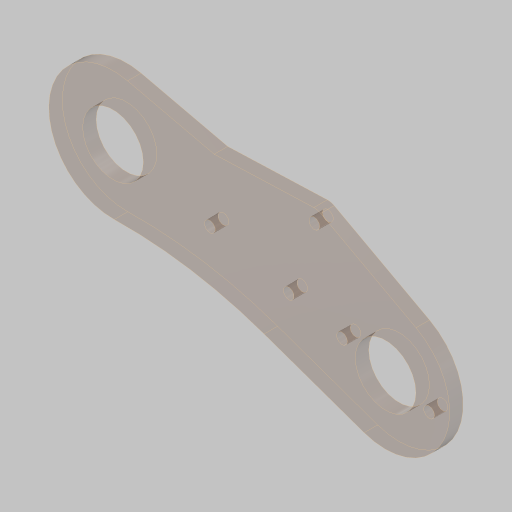
# Autodesk Inventor part: GP10-002
Saved by Autodesk Inventor 2023.5 (Build 275446000, 446)
## iProperties
Created: 2025-02-24
Part Number: GP10-002
Material: Polycarbonate, Smoke
Document SubType Name: Modeling
Designer: dlangdon
Density: 1.2 g/cm^3
Appearance: Polycarbonate - Smoked
Author: dlangdon
Autodesk Inventor part; units mm, degrees
ref_plane "YZ Plane" through (0, 0, 0) normal (1, 0, 0) x (0, 1, 0)
ref_plane "XZ Plane" through (0, 0, 0) normal (0, 1, 0) x (-1, 0, 0)
ref_plane "XY Plane" through (0, 0, 0) normal (0, 0, 1) x (1, 0, 0)
sketch "Sketch1" plane through (0, 0, 0) normal (0, 0, 1) x (1, 0, 0)
  circle A0 centre (71.842, 71.842) radius 50.8 construction
  circle A1 centre (-71.842, -71.842) radius 50.8 construction
  circle A2 centre (0, 0) radius 50.8 construction
  line L0 (-35.921, -35.921) -> (35.921, 35.921) construction
  line L1 (71.842, 71.842) -> (-71.842, -71.842) construction
  line L2 (-4.3707, 6.2419) -> (-4.3707, 50.6116) construction
  line L3 (-226.8798, -122.642) -> (638.5123, -122.642) construction
  circle A3 centre (147.8406, -65.492) radius 57.15 construction
  circle A4 centre (71.842, 71.842) radius 14.2621
  circle A5 centre (-71.842, -71.842) radius 14.2621
  circle A6 centre (-4.3707, 6.2419) radius 57.15 construction
  circle A7 centre (-71.842, -71.842) radius 30.1371 construction
  circle A8 centre (71.842, 71.842) radius 30.1371 construction
  circle A9 centre (-56.3286, 101.6778) radius 14.2621
  line L4 (-56.3286, 101.6778) -> (71.842, 71.842) construction
  circle A10 centre (71.842, 71.842) radius 14.3256 construction
  circle A11 centre (-71.842, -71.842) radius 14.3256 construction
  circle A12 centre (-78.675, 59.5778) radius 14.2621
  line L5 (-71.842, -71.842) -> (-78.675, 59.5778) construction
  circle A13 centre (-78.675, 59.5778) radius 23.8316 construction
  circle A14 centre (-56.3286, 101.6778) radius 23.8316 construction
  line L6 (14.7165, 60.1103) -> (61.7767, 43.4355)
  line L7 (-43.0113, -63.0652) -> (-59.0434, -10.4018)
  arc A15 (14.7165, 60.1103) -> (-59.0434, -10.4018) centre (-4.3707, 6.2419) ccw
  line L8 (-202.9564, 165.4321) -> (-177.9423, 161.0215)
  line L9 (-177.9423, 161.0215) -> (-204.4062, 10.9368) construction
  line L10 (-204.4062, 10.9368) -> (-229.4204, 15.3474) construction
  line L11 (-229.4204, 15.3474) -> (-202.9564, 165.4321) construction
  line L12 (-248.4004, -92.2937) -> (35.0702, -142.2772) construction
  line L13 (-201.8537, 171.6857) -> (161.0026, 107.7043) construction
  line L14 (-201.8537, 171.6857) -> (-248.4004, -92.2937) construction
  circle A16 centre (-147.7392, 94.6182) radius 31.75 construction
  line L15 (-77.4376, 35.7784) -> (-74.4797, -21.1106) construction
  line L16 (-190.4493, 163.2268) -> (-216.9133, 13.1421) construction
  line L17 (-193.206, 147.593) -> (-214.1566, 28.7759) construction
  circle A17 centre (-147.7392, 94.6182) radius 17.4625 construction
  circle A18 centre (-147.7392, 94.6182) radius 9.525
  circle A19 centre (-56.3286, 101.6778) radius 30.1816 construction
  line L18 (-202.9564, 165.4321) -> (-229.4204, 15.3474)
  arc A20 (61.7767, 43.4355) -> (78.6846, 101.1921) centre (71.842, 71.842) ccw
  arc A21 (-99.1524, -84.5852) -> (-43.0113, -63.0652) centre (-71.842, -71.842) ccw
  line L19 (-147.7392, 94.6182) -> (-131.3298, 100.5908) construction
  line L20 (-113.4287, 107.1063) -> (-182.0497, 82.1302) construction
  circle A22 centre (-182.0497, 82.1302) radius 4.7625 construction
  line L21 (0, 0) -> (-4.3707, 6.2419) construction
  circle A23 centre (71.842, 71.842) radius 28.6512 construction
  line L22 (62.334, 44.8145) -> (-61.0615, 88.2239) construction
  line L23 (75.2477, 100.2901) -> (-54.6333, 115.8388) construction
  line L24 (-177.9423, 161.0215) -> (78.6846, 101.1921)
  line L25 (-147.7392, 94.6182) -> (-125.7265, 22.8485) construction
  circle A24 centre (-125.7265, 22.8485) radius 31.75 construction
  circle A25 centre (-125.7265, 22.8485) radius 14.2621
  line L26 (-78.675, 59.5778) -> (-125.7265, 22.8485) construction
  circle A26 centre (-147.7392, 94.6182) radius 25.4 construction
  arc A27 (-99.1524, -84.5852) -> (-229.4204, 15.3474) centre (-260.2996, -159.7777) ccw
  circle A28 centre (-147.7392, 94.6182) radius 36.5125 construction
  line L27 (-180.8308, 110.0491) -> (-147.7392, 94.6182) construction
  arc A29 (-39.1085, 126.4648) -> (-49.6289, 131.1064) centre (-56.3286, 101.6778) ccw
  arc A30 (-38.1634, 52.3307) -> (-39.1085, 126.4648) centre (-65.0941, 89.0604) ccw
  arc A31 (14.7165, 60.1103) -> (-55.7287, 71.5022) centre (-51.7719, -127.535) ccw
  arc A32 (-49.6289, 131.1064) -> (-55.7287, 71.5022) centre (-56.3286, 101.6778) ccw
  line L28 (-10.7972, 91.0789) -> (26.3107, 82.4409) construction
  point P0 (-75.9587, 7.3339)
  point P1 (-203.6813, 88.1845)
  point P2 (-203.6813, 88.1845)
  point P3 (-144.7069, 111.8154)
  point P4 (-161.1163, 105.8429)
  point P5 (-164.1486, 88.6457)
  point P6 (-150.7715, 77.421)
  point P7 (-134.3622, 83.3936)
  point P8 (-123.871, 103.3056)
  point P9 (-143.3285, 119.6324)
  point P10 (-167.1967, 110.945)
  point P11 (-171.6074, 85.9309)
  point P12 (-152.1499, 69.6041)
  point P13 (-128.2817, 78.2914)
  point P14 (-160.2272, 128.9288)
  point P15 (-182.0497, 82.1302)
  point P16 (-135.2512, 60.3077)
  point P17 (-132.3084, 127.7098)
  point P18 (-163.1701, 61.5267)
  point P19 (-114.6476, 79.1874)
  point P20 (-49.4759, 131.0711)
  point P21 (7.7567, 86.7599)
  dimension "d7" = 101.6
  dimension "d18" = 47.6631
  dimension "d34" = 34.925
  dimension "d65" = 50.8
  dimension "d3" = 45
  dimension "d4" = 0
  dimension "d8" = 101.6
  dimension "d9" = 28.5242
  dimension "d10" = 101.6
  dimension "d11" = 114.3
  dimension "d12" = 114.3
  dimension "d13" = 15.875
  dimension "d14" = 15.875
  dimension "d15" = 131.5974
  dimension "d16" = 28.6512
  dimension "d17" = 131.5974
  dimension "d19" = 47.6631
  dimension "d22" = 25.4
  dimension "d23" = 152.4
  dimension "d26" = 268.0517
  dimension "d27" = 63.5
  dimension "d30" = 203.2
  dimension "d31" = 10
  dimension "d33" = 120.65
  dimension "d35" = 19.05
  dimension "d36" = 6.35
  dimension "d40" = 360
  dimension "d44" = 9.525
  dimension "d55" = 80
  dimension "d56" = 7.62
  dimension "d57" = 6.35
  dimension "d58" = 57.3024
  dimension "d59" = 63.5
  dimension "d60" = 75.0697
  dimension "d61" = 59.69
  dimension "d62" = 55
  dimension "d68" = 360
  dimension "d70" = 41.275
  dimension "d71" = 60
  dimension "d82" = 360
  dimension "d87" = 360
  dimension "d89" = 45
  dimension "d105" = 38.1
  constraints: 58 end point, 34 point on circle, 29 centre point, 27 coincident, 19 tangent, 9 midpoint, 6 equal radius, 6 point on line, 4 collinear, 4 parallel, 2 horizontal, 1 concentric, 1 perpendicular, 1 vertical, 39 other
  measures "d3" angle of L2 L0
  measures "d4" distance between parallel lines of L0 L1
  measures "d8" diameter of A2
  measures "d9" diameter of A4
  measures "d10" diameter of A0
  measures "d11" diameter of A3
  measures "d12" diameter of A6
  measures "d13" radial gap between concentric circles of A5 A7
  measures "d14" radial gap between concentric circles of A4 A8
  measures "d15" distance of L4.start L4.end
  measures "d16" diameter of A10
  measures "d17" distance of L5.start L5.end
  measures "d19" diameter of A14
  measures "d22" distance of L9.end L10.end
  measures "d23" distance of L10.end L8.start
  measures "d26" distance of L13.start L12.start
  measures "d27" diameter of A16
  measures "d30" distance from line of point (0, 0) L9
  measures "d31" angle of L3 L12
  measures "d33" distance of L17.start L17.end
  measures "d35" diameter of A18
  measures "d36" radial gap between concentric circles of A14 A19
  measures "d44" diameter of A22
  measures "d55" angle of L1 L21
  measures "d56" distance of L21.start L21.end
  measures "d57" distance between parallel lines of L13 L8
  measures "d58" diameter of A23
  measures "d59" diameter of A24
  measures "d60" distance of L19.start L25.end
  measures "d61" distance of L26.start L26.end
  measures "d62" angle of L15 L26
  measures "d70" distance from line of L9 L19.start
  measures "d71" angle of L9 L20
  measures "d89" angle of L20 L27
  measures "d105" distance of L28.start L28.end
extrude "Extrusion1" add sketch "Sketch1" along normal blind 6.35 contours A29 A30 A31 A32 | A31 A30 A29 L24 A20 L6
hole "Hole1" at (-193.206, 147.593, 0) at (-203.6813, 88.1845, 0) at (-214.1566, 28.7759, 0) at (-131.3298, 100.5908, 0) at (-144.7069, 111.8154, 0) at (-161.1163, 105.8429, 0) at (-164.1486, 88.6457, 0) at (-150.7715, 77.421, 0) at (-134.3622, 83.3936, 0) at (-113.4287, 107.1063, 0) at (-182.0497, 82.1302, 0) at (-152.1499, 69.6041, 0) at (-171.6074, 85.9309, 0) at (-167.1967, 110.945, 0) at (-143.3285, 119.6324, 0) at (-123.871, 103.3056, 0) at (-128.2817, 78.2914, 0) at (-75.9587, 7.3339, 0) at (-180.8308, 110.0491, 0) at (-132.3084, 127.7098, 0) at (-114.6476, 79.1874, 0) at (-163.1701, 61.5267, 0) at (-10.7972, 91.0789, 0) at (26.3107, 82.4409, 0) direction (0, 0, 1) diameter 5.1054 end through all clearance for "Flat Head Machine Screw (82)" size "#10" standard "Ansi Unified Screw Threads"
sketch "Sketch2" plane through (0, 0, 6.35) normal (0, 0, 1) x (1, 0, 0)
  line L0 (78.6846, 101.1921) -> (-49.4759, 131.0711) construction
  circle A0 centre (-56.3286, 101.6778) radius 14.2621 construction
  line L1 (-76.7997, 106.4431) -> (-35.8574, 96.9125) construction
  line L2 (51.3709, 76.6074) -> (92.3132, 67.0767) construction
  line L3 (-56.3286, 101.6778) -> (71.842, 71.842) construction
  arc A1 (-49.4759, 131.0711) -> (-55.7287, 71.5022) centre (-56.3286, 101.6778) ccw projected
  arc A2 (14.7165, 60.1103) -> (-55.7287, 71.5022) centre (-51.7719, -127.535) ccw projected
  line L4 (14.7165, 60.1103) -> (61.7767, 43.4355) projected
  arc A3 (61.7767, 43.4355) -> (78.6846, 101.1921) centre (71.842, 71.842) ccw projected
  point P0 (0, 0)
  constraints: 7 end point, 4 coincident, 3 collinear, 2 midpoint
hole "Hole2" at (92.3132, 67.0767, 6.35) at (51.3709, 76.6074, 6.35) direction (0, 0, -1) diameter 5.1054 end through all clearance for "Flat Head Machine Screw (82)" size "#10" standard "Ansi Unified Screw Threads"
sketch "Sketch3" plane through (0, 0, 6.35) normal (0, 0, 1) x (1, 0, 0)
  circle A0 centre (92.3132, 67.0767) radius 2.5527 construction
  circle A1 centre (51.3709, 76.6074) radius 2.5527 construction
  arc A2 (14.7165, 60.1103) -> (-55.7287, 71.5022) centre (-51.7719, -127.535) ccw construction
  line L0 (14.7165, 60.1103) -> (61.7767, 43.4355) construction
  arc A3 (61.7767, 43.4355) -> (78.6846, 101.1921) centre (71.842, 71.842) ccw construction
  line L1 (78.6846, 101.1921) -> (-49.4759, 131.0711) construction
  arc A4 (-49.4759, 131.0711) -> (-55.7287, 71.5022) centre (-56.3286, 101.6778) ccw construction
  circle A5 centre (71.842, 71.842) radius 14.2621 construction
  circle A6 centre (-56.3286, 101.6778) radius 14.2621 construction
  circle A7 centre (71.842, 71.842) radius 14.2621 construction
  line L2 (-56.3286, 101.6778) -> (71.842, 71.842) construction
  line L3 (30.0957, 81.5598) -> (38.3306, 116.936) construction
  line L4 (41.3443, 122.5253) -> (86.1452, 98.3687)
  arc A8 (61.7767, 43.4355) -> (78.6846, 101.1921) centre (71.842, 71.842) ccw construction
  line L5 (78.6846, 101.1921) -> (-49.4759, 131.0711) construction
  arc A9 (86.1452, 98.3687) -> (78.6846, 101.1921) centre (71.842, 71.842) ccw
  arc A10 (41.3443, 122.5253) -> (38.0994, 123.2818) centre (38.3306, 116.936) ccw
  arc A11 (36.8909, 110.7514) -> (36.9386, 110.7405) centre (38.3306, 116.936) ccw
  line L6 (38.0994, 123.2818) -> (-8.7442, 121.575)
  line L7 (78.6846, 101.1921) -> (-8.7442, 121.575)
  point P0 (0, 0)
  dimension "d90" = 42.8625
  dimension "d91" = 36.322
  dimension "d102" = 6.35
  dimension "d103" = 15.21
  dimension "d104" = 15.21
  constraints: 10 end point, 7 point on circle, 3 centre point, 3 point on line, 3 tangent, 2 coincident, 1 collinear, 1 perpendicular
  measures "d90" distance from line of L3 A3.centre
  measures "d91" distance of L3.start L3.end
  measures "d102" radius of A10
  measures "d103" angle of L1 L4
  measures "d104" angle of L1 L6
extrude "Extrusion2" add sketch "Sketch3" against normal up to surface (6.35 mm away)
sketch "Sketch4" plane through (0, 0, 6.35) normal (0, 0, 1) x (1, 0, 0)
  arc A0 (41.3443, 122.5253) -> (38.0994, 123.2818) centre (38.3306, 116.936) ccw construction
  point P0 (0, 0)
  constraints: 1 coincident
hole "Hole3" at (38.3306, 116.936, 6.35) direction (0, 0, -1) diameter 5.1054 end through all clearance for "Flat Head Machine Screw (82)" size "#10" standard "Ansi Unified Screw Threads"
body "Solid1"
